Autodesk Inventor part; units mm, degrees
(part 2 of 3)
  line L420 (-40.5392, 1.7059) -> (-40.4752, 1.693) construction
  line L421 (-40.4117, 1.6779) -> (-40.3487, 1.6594) construction
  line L422 (-40.3487, 1.6594) -> (-40.2906, 1.6288) construction
  arc A72 (-40.2906, 1.6288) -> (-40.3121, 0.9596) centre (0, 0) ccw
  arc A73 (-40.3121, 0.9596) -> (-40.3225, 0.2901) centre (0, 0) ccw
  spline S135 degree 4 poles (-40.5744, 0.225) (-40.5099, 0.2348) (-40.4457, 0.2469) (-40.382, 0.2624) (-40.3225, 0.2901) knots 1 1 1 1 1 2 2 2 2 2
  line L423 (-40.5744, 0.225) -> (-40.5099, 0.2348) construction
  line L424 (-40.5099, 0.2348) -> (-40.4457, 0.2469) construction
  line L425 (-40.4457, 0.2469) -> (-40.382, 0.2624) construction
  line L426 (-40.382, 0.2624) -> (-40.3225, 0.2901) construction
  line L427 (-42.9441, -4.507) -> (-41.7202, -3.9838) construction
  spline S136 degree 2 poles (-42.9441, -4.507) (-41.7202, -3.9838) (-40.4121, -3.6329) knots 1 1 1 2 2 2
  line L428 (-41.7202, -3.9838) -> (-40.4121, -3.6329) construction
  spline S137 degree 2 poles (-43.1484, -1.6505) (-41.8625, -1.9942) (-40.5178, -2.1553) knots 1 1 1 2 2 2
  line L429 (-43.1484, -1.6505) -> (-41.8625, -1.9942) construction
  line L430 (-41.8625, -1.9942) -> (-40.5178, -2.1553) construction
  line L431 (-40.4528, -2.1621) -> (-40.3882, -2.1711) construction
  spline S138 degree 4 poles (-40.5178, -2.1553) (-40.4528, -2.1621) (-40.3882, -2.1711) (-40.3237, -2.1835) (-40.263, -2.2084) knots 1 1 1 1 1 2 2 2 2 2
  line L432 (-40.5178, -2.1553) -> (-40.4528, -2.1621) construction
  line L433 (-40.3882, -2.1711) -> (-40.3237, -2.1835) construction
  line L434 (-40.3237, -2.1835) -> (-40.263, -2.2084) construction
  arc A74 (-40.263, -2.2084) -> (-40.2208, -2.8766) centre (0, 0) ccw
  arc A75 (-40.2208, -2.8766) -> (-40.1675, -3.5441) centre (0, 0) ccw
  spline S139 degree 4 poles (-40.4121, -3.6329) (-40.3488, -3.617) (-40.286, -3.5988) (-40.224, -3.5774) (-40.1675, -3.5441) knots 1 1 1 1 1 2 2 2 2 2
  line L435 (-40.4121, -3.6329) -> (-40.3488, -3.617) construction
  line L436 (-40.3488, -3.617) -> (-40.286, -3.5988) construction
  line L437 (-40.286, -3.5988) -> (-40.224, -3.5774) construction
  line L438 (-40.224, -3.5774) -> (-40.1675, -3.5441) construction
  line L439 (-42.3213, -8.5687) -> (-41.1526, -7.9315) construction
  spline S140 degree 2 poles (-42.3213, -8.5687) (-41.1526, -7.9315) (-39.8838, -7.4578) knots 1 1 1 2 2 2
  line L440 (-41.1526, -7.9315) -> (-39.8838, -7.4578) construction
  spline S141 degree 2 poles (-42.7962, -5.7445) (-41.4834, -5.9644) (-40.1294, -5.997) knots 1 1 1 2 2 2
  line L441 (-42.7962, -5.7445) -> (-41.4834, -5.9644) construction
  line L442 (-41.4834, -5.9644) -> (-40.1294, -5.997) construction
  line L443 (-40.0641, -5.9976) -> (-39.9989, -6.0004) construction
  spline S142 degree 4 poles (-40.1294, -5.997) (-40.0641, -5.9976) (-39.9989, -6.0004) (-39.9336, -6.0067) (-39.8708, -6.0257) knots 1 1 1 1 1 2 2 2 2 2
  line L444 (-40.1294, -5.997) -> (-40.0641, -5.9976) construction
  line L445 (-39.9989, -6.0004) -> (-39.9336, -6.0067) construction
  line L446 (-39.9336, -6.0067) -> (-39.8708, -6.0257) construction
  arc A76 (-39.8708, -6.0257) -> (-39.7652, -6.6869) centre (0, 0) ccw
  arc A77 (-39.7652, -6.6869) -> (-39.6487, -7.3462) centre (0, 0) ccw
  spline S143 degree 4 poles (-39.8838, -7.4578) (-39.8223, -7.436) (-39.7615, -7.412) (-39.7019, -7.3847) (-39.6487, -7.3462) knots 1 1 1 1 1 2 2 2 2 2
  line L447 (-39.8838, -7.4578) -> (-39.8223, -7.436) construction
  line L448 (-39.8223, -7.436) -> (-39.7615, -7.412) construction
  line L449 (-39.7615, -7.412) -> (-39.7019, -7.3847) construction
  line L450 (-39.7019, -7.3847) -> (-39.6487, -7.3462) construction
  line L451 (-41.3151, -12.5528) -> (-40.2124, -11.8074) construction
  spline S144 degree 2 poles (-41.3151, -12.5528) (-40.2124, -11.8074) (-38.9943, -11.2153) knots 1 1 1 2 2 2
  line L452 (-40.2124, -11.8074) -> (-38.9943, -11.2153) construction
  spline S145 degree 2 poles (-42.0563, -9.7866) (-40.7286, -9.8807) (-39.3777, -9.7844) knots 1 1 1 2 2 2
  line L453 (-42.0563, -9.7866) -> (-40.7286, -9.8807) construction
  line L454 (-40.7286, -9.8807) -> (-39.3777, -9.7844) construction
  line L455 (-39.3126, -9.7787) -> (-39.2474, -9.7754) construction
  spline S146 degree 4 poles (-39.3777, -9.7844) (-39.3126, -9.7787) (-39.2474, -9.7754) (-39.1818, -9.7754) (-39.1175, -9.7883) knots 1 1 1 1 1 2 2 2 2 2
  line L456 (-39.3777, -9.7844) -> (-39.3126, -9.7787) construction
  line L457 (-39.2474, -9.7754) -> (-39.1818, -9.7754) construction
  line L458 (-39.1818, -9.7754) -> (-39.1175, -9.7883) construction
  arc A78 (-39.1175, -9.7883) -> (-38.9496, -10.4365) centre (0, 0) ccw
  arc A79 (-38.9496, -10.4365) -> (-38.7709, -11.0818) centre (0, 0) ccw
  spline S147 degree 4 poles (-38.9943, -11.2153) (-38.9351, -11.1877) (-38.8769, -11.158) (-38.8201, -11.1252) (-38.7709, -11.0818) knots 1 1 1 1 1 2 2 2 2 2
  line L459 (-38.9943, -11.2153) -> (-38.9351, -11.1877) construction
  line L460 (-38.9351, -11.1877) -> (-38.8769, -11.158) construction
  line L461 (-38.8769, -11.158) -> (-38.8201, -11.1252) construction
  line L462 (-38.8201, -11.1252) -> (-38.7709, -11.0818) construction
  line L463 (-39.9348, -16.4232) -> (-38.9079, -15.5764) construction
  spline S148 degree 2 poles (-39.9348, -16.4232) (-38.9079, -15.5764) (-37.7516, -14.8711) knots 1 1 1 2 2 2
  line L464 (-38.9079, -15.5764) -> (-37.7516, -14.8711) construction
  spline S149 degree 2 poles (-40.9356, -13.7399) (-39.605, -13.7074) (-38.2693, -13.4832) knots 1 1 1 2 2 2
  line L465 (-40.9356, -13.7399) -> (-39.605, -13.7074) construction
  line L466 (-39.605, -13.7074) -> (-38.2693, -13.4832) construction
  line L467 (-38.2051, -13.4714) -> (-38.1405, -13.4618) construction
  spline S150 degree 4 poles (-38.2693, -13.4832) (-38.2051, -13.4714) (-38.1405, -13.4618) (-38.0752, -13.4556) (-38.0099, -13.4624) knots 1 1 1 1 1 2 2 2 2 2
  line L468 (-38.2693, -13.4832) -> (-38.2051, -13.4714) construction
  line L469 (-38.1405, -13.4618) -> (-38.0752, -13.4556) construction
  line L470 (-38.0752, -13.4556) -> (-38.0099, -13.4624) construction
  arc A80 (-38.0099, -13.4624) -> (-37.7811, -14.0916) centre (0, 0) ccw
  arc A81 (-37.7811, -14.0916) -> (-37.5419, -14.717) centre (0, 0) ccw
  spline S151 degree 4 poles (-37.7516, -14.8711) (-37.6953, -14.838) (-37.6403, -14.8029) (-37.5868, -14.7649) (-37.5419, -14.717) knots 1 1 1 1 1 2 2 2 2 2
  line L471 (-37.7516, -14.8711) -> (-37.6953, -14.838) construction
  line L472 (-37.6953, -14.838) -> (-37.6403, -14.8029) construction
  line L473 (-37.6403, -14.8029) -> (-37.5868, -14.7649) construction
  line L474 (-37.5868, -14.7649) -> (-37.5419, -14.717) construction
  line L475 (-38.1929, -20.1449) -> (-37.2511, -19.2043) construction
  spline S152 degree 2 poles (-38.1929, -20.1449) (-37.2511, -19.2043) (-36.1671, -18.3923) knots 1 1 1 2 2 2
  line L476 (-37.2511, -19.2043) -> (-36.1671, -18.3923) construction
  spline S153 degree 2 poles (-39.4442, -17.5689) (-38.1227, -17.41) (-36.8144, -17.0599) knots 1 1 1 2 2 2
  line L477 (-39.4442, -17.5689) -> (-38.1227, -17.41) construction
  line L478 (-38.1227, -17.41) -> (-36.8144, -17.0599) construction
  line L479 (-36.7515, -17.042) -> (-36.6882, -17.0263) construction
  spline S154 degree 4 poles (-36.8144, -17.0599) (-36.7515, -17.042) (-36.6882, -17.0263) (-36.6237, -17.0139) (-36.5581, -17.0145) knots 1 1 1 1 1 2 2 2 2 2
  line L480 (-36.8144, -17.0599) -> (-36.7515, -17.042) construction
  line L481 (-36.6882, -17.0263) -> (-36.6237, -17.0139) construction
  line L482 (-36.6237, -17.0139) -> (-36.5581, -17.0145) construction
  arc A82 (-36.5581, -17.0145) -> (-36.2706, -17.6192) centre (0, 0) ccw
  arc A83 (-36.2706, -17.6192) -> (-35.973, -18.219) centre (0, 0) ccw
  spline S155 degree 4 poles (-36.1671, -18.3923) (-36.1142, -18.354) (-36.0627, -18.3138) (-36.0131, -18.2709) (-35.973, -18.219) knots 1 1 1 1 1 2 2 2 2 2
  line L483 (-36.1671, -18.3923) -> (-36.1142, -18.354) construction
  line L484 (-36.1142, -18.354) -> (-36.0627, -18.3138) construction
  line L485 (-36.0627, -18.3138) -> (-36.0131, -18.2709) construction
  line L486 (-36.0131, -18.2709) -> (-35.973, -18.219) construction
  line L487 (-36.1051, -23.6841) -> (-35.2569, -22.6583) construction
  spline S156 degree 2 poles (-36.1051, -23.6841) (-35.2569, -22.6583) (-34.255, -21.7469) knots 1 1 1 2 2 2
  line L488 (-35.2569, -22.6583) -> (-34.255, -21.7469) construction
  spline S157 degree 2 poles (-37.5956, -21.2388) (-36.2951, -20.955) (-35.026, -20.4821) knots 1 1 1 2 2 2
  line L489 (-37.5956, -21.2388) -> (-36.2951, -20.955) construction
  line L490 (-36.2951, -20.955) -> (-35.026, -20.4821) construction
  line L491 (-34.9652, -20.4583) -> (-34.9036, -20.4367) construction
  spline S158 degree 4 poles (-35.026, -20.4821) (-34.9652, -20.4583) (-34.9036, -20.4367) (-34.8406, -20.4182) (-34.7752, -20.4125) knots 1 1 1 1 1 2 2 2 2 2
  line L492 (-35.026, -20.4821) -> (-34.9652, -20.4583) construction
  line L493 (-34.9036, -20.4367) -> (-34.8406, -20.4182) construction
  line L494 (-34.8406, -20.4182) -> (-34.7752, -20.4125) construction
  arc A84 (-34.7752, -20.4125) -> (-34.4315, -20.9871) centre (0, 0) ccw
  arc A85 (-34.4315, -20.9871) -> (-34.0783, -21.5559) centre (0, 0) ccw
  spline S159 degree 4 poles (-34.255, -21.7469) (-34.206, -21.7038) (-34.1586, -21.6589) (-34.1133, -21.6114) (-34.0783, -21.5559) knots 1 1 1 1 1 2 2 2 2 2
  line L495 (-34.255, -21.7469) -> (-34.206, -21.7038) construction
  line L496 (-34.206, -21.7038) -> (-34.1586, -21.6589) construction
  line L497 (-34.1586, -21.6589) -> (-34.1133, -21.6114) construction
  line L498 (-34.1133, -21.6114) -> (-34.0783, -21.5559) construction
  line L499 (-33.6903, -27.0089) -> (-32.9435, -25.907) construction
  spline S160 degree 2 poles (-33.6903, -27.0089) (-32.9435, -25.907) (-32.0327, -24.9046) knots 1 1 1 2 2 2
  line L500 (-32.9435, -25.907) -> (-32.0327, -24.9046) construction
  spline S161 degree 2 poles (-35.4065, -24.7163) (-34.1389, -24.3102) (-32.9205, -23.7188) knots 1 1 1 2 2 2
  line L501 (-35.4065, -24.7163) -> (-34.1389, -24.3102) construction
  line L502 (-34.1389, -24.3102) -> (-32.9205, -23.7188) construction
  line L503 (-32.8622, -23.6893) -> (-32.8029, -23.6619) construction
  spline S162 degree 4 poles (-32.9205, -23.7188) (-32.8622, -23.6893) (-32.8029, -23.6619) (-32.742, -23.6376) (-32.6774, -23.6257) knots 1 1 1 1 1 2 2 2 2 2
  line L504 (-32.9205, -23.7188) -> (-32.8622, -23.6893) construction
  line L505 (-32.8029, -23.6619) -> (-32.742, -23.6376) construction
  line L506 (-32.742, -23.6376) -> (-32.6774, -23.6257) construction
  arc A86 (-32.6774, -23.6257) -> (-32.2807, -24.165) centre (0, 0) ccw
  arc A87 (-32.2807, -24.165) -> (-31.875, -24.6977) centre (0, 0) ccw
  spline S163 degree 4 poles (-32.0327, -24.9046) (-31.9881, -24.857) (-31.9451, -24.8078) (-31.9046, -24.7562) (-31.875, -24.6977) knots 1 1 1 1 1 2 2 2 2 2
  line L507 (-32.0327, -24.9046) -> (-31.9881, -24.857) construction
  line L508 (-31.9881, -24.857) -> (-31.9451, -24.8078) construction
  line L509 (-31.9451, -24.8078) -> (-31.9046, -24.7562) construction
  line L510 (-31.9046, -24.7562) -> (-31.875, -24.6977) construction
  line L511 (-30.9703, -30.089) -> (-30.3317, -28.9212) construction
  spline S164 degree 2 poles (-30.9703, -30.089) (-30.3317, -28.9212) (-29.5204, -27.8367) knots 1 1 1 2 2 2
  line L512 (-30.3317, -28.9212) -> (-29.5204, -27.8367) construction
  spline S165 degree 2 poles (-32.8967, -27.97) (-31.6735, -27.4452) (-30.5168, -26.7406) knots 1 1 1 2 2 2
  line L513 (-32.8967, -27.97) -> (-31.6735, -27.4452) construction
  line L514 (-31.6735, -27.4452) -> (-30.5168, -26.7406) construction
  line L515 (-30.4616, -26.7058) -> (-30.4051, -26.6729) construction
  spline S166 degree 4 poles (-30.5168, -26.7406) (-30.4616, -26.7058) (-30.4051, -26.6729) (-30.3468, -26.6429) (-30.2837, -26.6249) knots 1 1 1 1 1 2 2 2 2 2
  line L516 (-30.5168, -26.7406) -> (-30.4616, -26.7058) construction
  line L517 (-30.4051, -26.6729) -> (-30.3468, -26.6429) construction
  line L518 (-30.3468, -26.6429) -> (-30.2837, -26.6249) construction
  arc A88 (-30.2837, -26.6249) -> (-29.8375, -27.1241) centre (0, 0) ccw
  arc A89 (-29.8375, -27.1241) -> (-29.383, -27.6157) centre (0, 0) ccw
  spline S167 degree 4 poles (-29.5204, -27.8367) (-29.4804, -27.7851) (-29.4423, -27.732) (-29.4069, -27.6768) (-29.383, -27.6157) knots 1 1 1 1 1 2 2 2 2 2
  line L519 (-29.5204, -27.8367) -> (-29.4804, -27.7851) construction
  line L520 (-29.4804, -27.7851) -> (-29.4423, -27.732) construction
  line L521 (-29.4423, -27.732) -> (-29.4069, -27.6768) construction
  line L522 (-29.4069, -27.6768) -> (-29.383, -27.6157) construction
  line L523 (-27.97, -32.8967) -> (-27.4452, -31.6735) construction
  spline S168 degree 2 poles (-27.97, -32.8967) (-27.4452, -31.6735) (-26.7406, -30.5168) knots 1 1 1 2 2 2
  line L524 (-27.4452, -31.6735) -> (-26.7406, -30.5168) construction
  spline S169 degree 2 poles (-30.089, -30.9703) (-28.9212, -30.3317) (-27.8367, -29.5204) knots 1 1 1 2 2 2
  line L525 (-30.089, -30.9703) -> (-28.9212, -30.3317) construction
  line L526 (-28.9212, -30.3317) -> (-27.8367, -29.5204) construction
  line L527 (-27.7851, -29.4804) -> (-27.732, -29.4423) construction
  spline S170 degree 4 poles (-27.8367, -29.5204) (-27.7851, -29.4804) (-27.732, -29.4423) (-27.6768, -29.4069) (-27.6157, -29.383) knots 1 1 1 1 1 2 2 2 2 2
  line L528 (-27.8367, -29.5204) -> (-27.7851, -29.4804) construction
  line L529 (-27.732, -29.4423) -> (-27.6768, -29.4069) construction
  line L530 (-27.6768, -29.4069) -> (-27.6157, -29.383) construction
  arc A90 (-27.6157, -29.383) -> (-27.1241, -29.8375) centre (0, 0) ccw
  arc A91 (-27.1241, -29.8375) -> (-26.6249, -30.2837) centre (0, 0) ccw
  spline S171 degree 4 poles (-26.7406, -30.5168) (-26.7058, -30.4616) (-26.6729, -30.4051) (-26.6429, -30.3468) (-26.6249, -30.2837) knots 1 1 1 1 1 2 2 2 2 2
  line L531 (-26.7406, -30.5168) -> (-26.7058, -30.4616) construction
  line L532 (-26.7058, -30.4616) -> (-26.6729, -30.4051) construction
  line L533 (-26.6729, -30.4051) -> (-26.6429, -30.3468) construction
  line L534 (-26.6429, -30.3468) -> (-26.6249, -30.2837) construction
  line L535 (-24.7163, -35.4065) -> (-24.3102, -34.1389) construction
  spline S172 degree 2 poles (-24.7163, -35.4065) (-24.3102, -34.1389) (-23.7188, -32.9205) knots 1 1 1 2 2 2
  line L536 (-24.3102, -34.1389) -> (-23.7188, -32.9205) construction
  spline S173 degree 2 poles (-27.0089, -33.6903) (-25.907, -32.9435) (-24.9046, -32.0327) knots 1 1 1 2 2 2
  line L537 (-27.0089, -33.6903) -> (-25.907, -32.9435) construction
  line L538 (-25.907, -32.9435) -> (-24.9046, -32.0327) construction
  line L539 (-24.857, -31.9881) -> (-24.8078, -31.9451) construction
  spline S174 degree 4 poles (-24.9046, -32.0327) (-24.857, -31.9881) (-24.8078, -31.9451) (-24.7562, -31.9046) (-24.6977, -31.875) knots 1 1 1 1 1 2 2 2 2 2
  line L540 (-24.9046, -32.0327) -> (-24.857, -31.9881) construction
  line L541 (-24.8078, -31.9451) -> (-24.7562, -31.9046) construction
  line L542 (-24.7562, -31.9046) -> (-24.6977, -31.875) construction
  arc A92 (-24.6977, -31.875) -> (-24.165, -32.2807) centre (0, 0) ccw
  arc A93 (-24.165, -32.2807) -> (-23.6257, -32.6774) centre (0, 0) ccw
  spline S175 degree 4 poles (-23.7188, -32.9205) (-23.6893, -32.8622) (-23.6619, -32.8029) (-23.6376, -32.742) (-23.6257, -32.6774) knots 1 1 1 1 1 2 2 2 2 2
  line L543 (-23.7188, -32.9205) -> (-23.6893, -32.8622) construction
  line L544 (-23.6893, -32.8622) -> (-23.6619, -32.8029) construction
  line L545 (-23.6619, -32.8029) -> (-23.6376, -32.742) construction
  line L546 (-23.6376, -32.742) -> (-23.6257, -32.6774) construction
  line L547 (-21.2388, -37.5956) -> (-20.955, -36.2951) construction
  spline S176 degree 2 poles (-21.2388, -37.5956) (-20.955, -36.2951) (-20.4821, -35.026) knots 1 1 1 2 2 2
  line L548 (-20.955, -36.2951) -> (-20.4821, -35.026) construction
  spline S177 degree 2 poles (-23.6841, -36.1051) (-22.6583, -35.2569) (-21.7469, -34.255) knots 1 1 1 2 2 2
  line L549 (-23.6841, -36.1051) -> (-22.6583, -35.2569) construction
  line L550 (-22.6583, -35.2569) -> (-21.7469, -34.255) construction
  line L551 (-21.7038, -34.206) -> (-21.6589, -34.1586) construction
  spline S178 degree 4 poles (-21.7469, -34.255) (-21.7038, -34.206) (-21.6589, -34.1586) (-21.6114, -34.1133) (-21.5559, -34.0783) knots 1 1 1 1 1 2 2 2 2 2
  line L552 (-21.7469, -34.255) -> (-21.7038, -34.206) construction
  line L553 (-21.6589, -34.1586) -> (-21.6114, -34.1133) construction
  line L554 (-21.6114, -34.1133) -> (-21.5559, -34.0783) construction
  arc A94 (-21.5559, -34.0783) -> (-20.9871, -34.4315) centre (0, 0) ccw
  arc A95 (-20.9871, -34.4315) -> (-20.4125, -34.7752) centre (0, 0) ccw
  spline S179 degree 4 poles (-20.4821, -35.026) (-20.4583, -34.9652) (-20.4367, -34.9036) (-20.4182, -34.8406) (-20.4125, -34.7752) knots 1 1 1 1 1 2 2 2 2 2
  line L555 (-20.4821, -35.026) -> (-20.4583, -34.9652) construction
  line L556 (-20.4583, -34.9652) -> (-20.4367, -34.9036) construction
  line L557 (-20.4367, -34.9036) -> (-20.4182, -34.8406) construction
  line L558 (-20.4182, -34.8406) -> (-20.4125, -34.7752) construction
  line L559 (-17.5689, -39.4442) -> (-17.41, -38.1227) construction
  spline S180 degree 2 poles (-17.5689, -39.4442) (-17.41, -38.1227) (-17.0599, -36.8144) knots 1 1 1 2 2 2
  line L560 (-17.41, -38.1227) -> (-17.0599, -36.8144) construction
  spline S181 degree 2 poles (-20.1449, -38.1929) (-19.2043, -37.2511) (-18.3923, -36.1671) knots 1 1 1 2 2 2
  line L561 (-20.1449, -38.1929) -> (-19.2043, -37.2511) construction
  line L562 (-19.2043, -37.2511) -> (-18.3923, -36.1671) construction
  line L563 (-18.354, -36.1142) -> (-18.3138, -36.0627) construction
  spline S182 degree 4 poles (-18.3923, -36.1671) (-18.354, -36.1142) (-18.3138, -36.0627) (-18.2709, -36.0131) (-18.219, -35.973) knots 1 1 1 1 1 2 2 2 2 2
  line L564 (-18.3923, -36.1671) -> (-18.354, -36.1142) construction
  line L565 (-18.3138, -36.0627) -> (-18.2709, -36.0131) construction
  line L566 (-18.2709, -36.0131) -> (-18.219, -35.973) construction
  arc A96 (-18.219, -35.973) -> (-17.6192, -36.2706) centre (0, 0) ccw
  arc A97 (-17.6192, -36.2706) -> (-17.0145, -36.5581) centre (0, 0) ccw
  spline S183 degree 4 poles (-17.0599, -36.8144) (-17.042, -36.7515) (-17.0263, -36.6882) (-17.0139, -36.6237) (-17.0145, -36.5581) knots 1 1 1 1 1 2 2 2 2 2
  line L567 (-17.0599, -36.8144) -> (-17.042, -36.7515) construction
  line L568 (-17.042, -36.7515) -> (-17.0263, -36.6882) construction
  line L569 (-17.0263, -36.6882) -> (-17.0139, -36.6237) construction
  line L570 (-17.0139, -36.6237) -> (-17.0145, -36.5581) construction
  line L571 (-13.7399, -40.9356) -> (-13.7074, -39.605) construction
  spline S184 degree 2 poles (-13.7399, -40.9356) (-13.7074, -39.605) (-13.4832, -38.2693) knots 1 1 1 2 2 2
  line L572 (-13.7074, -39.605) -> (-13.4832, -38.2693) construction
  spline S185 degree 2 poles (-16.4232, -39.9348) (-15.5764, -38.9079) (-14.8711, -37.7516) knots 1 1 1 2 2 2
  line L573 (-16.4232, -39.9348) -> (-15.5764, -38.9079) construction
  line L574 (-15.5764, -38.9079) -> (-14.8711, -37.7516) construction
  line L575 (-14.838, -37.6953) -> (-14.8029, -37.6403) construction
  spline S186 degree 4 poles (-14.8711, -37.7516) (-14.838, -37.6953) (-14.8029, -37.6403) (-14.7649, -37.5868) (-14.717, -37.5419) knots 1 1 1 1 1 2 2 2 2 2
  line L576 (-14.8711, -37.7516) -> (-14.838, -37.6953) construction
  line L577 (-14.8029, -37.6403) -> (-14.7649, -37.5868) construction
  line L578 (-14.7649, -37.5868) -> (-14.717, -37.5419) construction
  arc A98 (-14.717, -37.5419) -> (-14.0916, -37.7811) centre (0, 0) ccw
  arc A99 (-14.0916, -37.7811) -> (-13.4624, -38.0099) centre (0, 0) ccw
  spline S187 degree 4 poles (-13.4832, -38.2693) (-13.4714, -38.2051) (-13.4618, -38.1405) (-13.4556, -38.0752) (-13.4624, -38.0099) knots 1 1 1 1 1 2 2 2 2 2
  line L579 (-13.4832, -38.2693) -> (-13.4714, -38.2051) construction
  line L580 (-13.4714, -38.2051) -> (-13.4618, -38.1405) construction
  line L581 (-13.4618, -38.1405) -> (-13.4556, -38.0752) construction
  line L582 (-13.4556, -38.0752) -> (-13.4624, -38.0099) construction
  line L583 (-9.7866, -42.0563) -> (-9.8807, -40.7286) construction
  spline S188 degree 2 poles (-9.7866, -42.0563) (-9.8807, -40.7286) (-9.7844, -39.3777) knots 1 1 1 2 2 2
  line L584 (-9.8807, -40.7286) -> (-9.7844, -39.3777) construction
  spline S189 degree 2 poles (-12.5528, -41.3151) (-11.8074, -40.2124) (-11.2153, -38.9943) knots 1 1 1 2 2 2
  line L585 (-12.5528, -41.3151) -> (-11.8074, -40.2124) construction
  line L586 (-11.8074, -40.2124) -> (-11.2153, -38.9943) construction
  line L587 (-11.1877, -38.9351) -> (-11.158, -38.8769) construction
  spline S190 degree 4 poles (-11.2153, -38.9943) (-11.1877, -38.9351) (-11.158, -38.8769) (-11.1252, -38.8201) (-11.0818, -38.7709) knots 1 1 1 1 1 2 2 2 2 2
  line L588 (-11.2153, -38.9943) -> (-11.1877, -38.9351) construction
  line L589 (-11.158, -38.8769) -> (-11.1252, -38.8201) construction
  line L590 (-11.1252, -38.8201) -> (-11.0818, -38.7709) construction
  arc A100 (-11.0818, -38.7709) -> (-10.4365, -38.9496) centre (0, 0) ccw
  arc A101 (-10.4365, -38.9496) -> (-9.7883, -39.1175) centre (0, 0) ccw
  spline S191 degree 4 poles (-9.7844, -39.3777) (-9.7787, -39.3126) (-9.7754, -39.2474) (-9.7754, -39.1818) (-9.7883, -39.1175) knots 1 1 1 1 1 2 2 2 2 2
  line L591 (-9.7844, -39.3777) -> (-9.7787, -39.3126) construction
  line L592 (-9.7787, -39.3126) -> (-9.7754, -39.2474) construction
  line L593 (-9.7754, -39.2474) -> (-9.7754, -39.1818) construction
  line L594 (-9.7754, -39.1818) -> (-9.7883, -39.1175) construction
  line L595 (-5.7445, -42.7962) -> (-5.9644, -41.4834) construction
  spline S192 degree 2 poles (-5.7445, -42.7962) (-5.9644, -41.4834) (-5.997, -40.1294) knots 1 1 1 2 2 2
  line L596 (-5.9644, -41.4834) -> (-5.997, -40.1294) construction
  spline S193 degree 2 poles (-8.5687, -42.3213) (-7.9315, -41.1526) (-7.4578, -39.8838) knots 1 1 1 2 2 2
  line L597 (-8.5687, -42.3213) -> (-7.9315, -41.1526) construction
  line L598 (-7.9315, -41.1526) -> (-7.4578, -39.8838) construction
  line L599 (-7.436, -39.8223) -> (-7.412, -39.7615) construction
  spline S194 degree 4 poles (-7.4578, -39.8838) (-7.436, -39.8223) (-7.412, -39.7615) (-7.3847, -39.7019) (-7.3462, -39.6487) knots 1 1 1 1 1 2 2 2 2 2
  line L600 (-7.4578, -39.8838) -> (-7.436, -39.8223) construction
  line L601 (-7.412, -39.7615) -> (-7.3847, -39.7019) construction
  line L602 (-7.3847, -39.7019) -> (-7.3462, -39.6487) construction
  arc A102 (-7.3462, -39.6487) -> (-6.6869, -39.7652) centre (0, 0) ccw
  arc A103 (-6.6869, -39.7652) -> (-6.0257, -39.8708) centre (0, 0) ccw
  spline S195 degree 4 poles (-5.997, -40.1294) (-5.9976, -40.0641) (-6.0004, -39.9989) (-6.0067, -39.9336) (-6.0257, -39.8708) knots 1 1 1 1 1 2 2 2 2 2
  line L603 (-5.997, -40.1294) -> (-5.9976, -40.0641) construction
  line L604 (-5.9976, -40.0641) -> (-6.0004, -39.9989) construction
  line L605 (-6.0004, -39.9989) -> (-6.0067, -39.9336) construction
  line L606 (-6.0067, -39.9336) -> (-6.0257, -39.8708) construction
  line L607 (-1.6505, -43.1484) -> (-1.9942, -41.8625) construction
  spline S196 degree 2 poles (-1.6505, -43.1484) (-1.9942, -41.8625) (-2.1553, -40.5178) knots 1 1 1 2 2 2
  line L608 (-1.9942, -41.8625) -> (-2.1553, -40.5178) construction
  spline S197 degree 2 poles (-4.507, -42.9441) (-3.9838, -41.7202) (-3.6329, -40.4121) knots 1 1 1 2 2 2
  line L609 (-4.507, -42.9441) -> (-3.9838, -41.7202) construction
  line L610 (-3.9838, -41.7202) -> (-3.6329, -40.4121) construction
  line L611 (-3.617, -40.3488) -> (-3.5988, -40.286) construction
  spline S198 degree 4 poles (-3.6329, -40.4121) (-3.617, -40.3488) (-3.5988, -40.286) (-3.5774, -40.224) (-3.5441, -40.1675) knots 1 1 1 1 1 2 2 2 2 2
  line L612 (-3.6329, -40.4121) -> (-3.617, -40.3488) construction
  line L613 (-3.5988, -40.286) -> (-3.5774, -40.224) construction
  line L614 (-3.5774, -40.224) -> (-3.5441, -40.1675) construction
  arc A104 (-3.5441, -40.1675) -> (-2.8766, -40.2208) centre (0, 0) ccw
  arc A105 (-2.8766, -40.2208) -> (-2.2084, -40.263) centre (0, 0) ccw
  spline S199 degree 4 poles (-2.1553, -40.5178) (-2.1621, -40.4528) (-2.1711, -40.3882) (-2.1835, -40.3237) (-2.2084, -40.263) knots 1 1 1 1 1 2 2 2 2 2
  line L615 (-2.1553, -40.5178) -> (-2.1621, -40.4528) construction
  line L616 (-2.1621, -40.4528) -> (-2.1711, -40.3882) construction
  line L617 (-2.1711, -40.3882) -> (-2.1835, -40.3237) construction
  line L618 (-2.1835, -40.3237) -> (-2.2084, -40.263) construction
  line L619 (2.4585, -43.11) -> (1.9942, -41.8625) construction
  spline S200 degree 2 poles (2.4585, -43.11) (1.9942, -41.8625) (1.7059, -40.5392) knots 1 1 1 2 2 2
  line L620 (1.9942, -41.8625) -> (1.7059, -40.5392) construction
  spline S201 degree 2 poles (-0.4045, -43.1781) (0, -41.91) (0.225, -40.5744) knots 1 1 1 2 2 2
  line L621 (-0.4045, -43.1781) -> (0, -41.91) construction
  line L622 (0, -41.91) -> (0.225, -40.5744) construction
  line L623 (0.2348, -40.5099) -> (0.2469, -40.4457) construction
  spline S202 degree 4 poles (0.225, -40.5744) (0.2348, -40.5099) (0.2469, -40.4457) (0.2624, -40.382) (0.2901, -40.3225) knots 1 1 1 1 1 2 2 2 2 2
  line L624 (0.225, -40.5744) -> (0.2348, -40.5099) construction
  line L625 (0.2469, -40.4457) -> (0.2624, -40.382) construction
  line L626 (0.2624, -40.382) -> (0.2901, -40.3225) construction
  arc A106 (0.2901, -40.3225) -> (0.9596, -40.3121) centre (0, 0) ccw
  arc A107 (0.9596, -40.3121) -> (1.6288, -40.2906) centre (0, 0) ccw
  spline S203 degree 4 poles (1.7059, -40.5392) (1.693, -40.4752) (1.6779, -40.4117) (1.6594, -40.3487) (1.6288, -40.2906) knots 1 1 1 1 1 2 2 2 2 2
  line L627 (1.7059, -40.5392) -> (1.693, -40.4752) construction
  line L628 (1.693, -40.4752) -> (1.6779, -40.4117) construction
  line L629 (1.6779, -40.4117) -> (1.6594, -40.3487) construction
  line L630 (1.6594, -40.3487) -> (1.6288, -40.2906) construction
  line L631 (6.5452, -42.6811) -> (5.9644, -41.4834) construction
  spline S204 degree 2 poles (6.5452, -42.6811) (5.9644, -41.4834) (5.5517, -40.1935) knots 1 1 1 2 2 2
  line L632 (5.9644, -41.4834) -> (5.5517, -40.1935) construction
  spline S205 degree 2 poles (3.7017, -43.021) (3.9838, -41.7202) (4.0808, -40.3693) knots 1 1 1 2 2 2
  line L633 (3.7017, -43.021) -> (3.9838, -41.7202) construction
  line L634 (3.9838, -41.7202) -> (4.0808, -40.3693) construction
  line L635 (4.0844, -40.3041) -> (4.0904, -40.2391) construction
  spline S206 degree 4 poles (4.0808, -40.3693) (4.0844, -40.3041) (4.0904, -40.2391) (4.0997, -40.1742) (4.1217, -40.1123) knots 1 1 1 1 1 2 2 2 2 2
  line L636 (4.0808, -40.3693) -> (4.0844, -40.3041) construction
  line L637 (4.0904, -40.2391) -> (4.0997, -40.1742) construction
  line L638 (4.0997, -40.1742) -> (4.1217, -40.1123) construction
  arc A108 (4.1217, -40.1123) -> (4.7872, -40.0384) centre (0, 0) ccw
  arc A109 (4.7872, -40.0384) -> (5.4513, -39.9534) centre (0, 0) ccw
  spline S207 degree 4 poles (5.5517, -40.1935) (5.5328, -40.131) (5.5116, -40.0692) (5.4872, -40.0083) (5.4513, -39.9534) knots 1 1 1 1 1 2 2 2 2 2
  line L639 (5.5517, -40.1935) -> (5.5328, -40.131) construction
  line L640 (5.5328, -40.131) -> (5.5116, -40.0692) construction
  line L641 (5.5116, -40.0692) -> (5.4872, -40.0083) construction
  line L642 (5.4872, -40.0083) -> (5.4513, -39.9534) construction
  line L643 (10.5727, -41.8656) -> (9.8807, -40.7286) construction
  spline S208 degree 2 poles (10.5727, -41.8656) (9.8807, -40.7286) (9.3471, -39.4838) knots 1 1 1 2 2 2
  line L644 (9.8807, -40.7286) -> (9.3471, -39.4838) construction
  spline S209 degree 2 poles (7.7743, -42.4744) (7.9315, -41.1526) (7.8997, -39.7986) knots 1 1 1 2 2 2
  line L645 (7.7743, -42.4744) -> (7.9315, -41.1526) construction
  line L646 (7.9315, -41.1526) -> (7.8997, -39.7986) construction
  line L647 (7.8971, -39.7334) -> (7.8968, -39.6681) construction
  spline S210 degree 4 poles (7.8997, -39.7986) (7.8971, -39.7334) (7.8968, -39.6681) (7.9, -39.6025) (7.916, -39.5389) knots 1 1 1 1 1 2 2 2 2 2
  line L648 (7.8997, -39.7986) -> (7.8971, -39.7334) construction
  line L649 (7.8968, -39.6681) -> (7.9, -39.6025) construction
  line L650 (7.9, -39.6025) -> (7.916, -39.5389) construction
  arc A110 (7.916, -39.5389) -> (8.5714, -39.402) centre (0, 0) ccw
  arc A111 (8.5714, -39.402) -> (9.2244, -39.2543) centre (0, 0) ccw
  spline S211 degree 4 poles (9.3471, -39.4838) (9.3224, -39.4233) (9.2955, -39.3638) (9.2654, -39.3055) (9.2244, -39.2543) knots 1 1 1 1 1 2 2 2 2 2
  line L651 (9.3471, -39.4838) -> (9.3224, -39.4233) construction
  line L652 (9.3224, -39.4233) -> (9.2955, -39.3638) construction
  line L653 (9.2955, -39.3638) -> (9.2654, -39.3055) construction
  line L654 (9.2654, -39.3055) -> (9.2244, -39.2543) construction
  line L655 (14.5044, -40.6711) -> (13.7074, -39.605) construction
  spline S212 degree 2 poles (14.5044, -40.6711) (13.7074, -39.605) (13.058, -38.4165) knots 1 1 1 2 2 2
  line L656 (13.7074, -39.605) -> (13.058, -38.4165) construction
  spline S213 degree 2 poles (11.7766, -41.543) (11.8074, -40.2124) (11.647, -38.8675) knots 1 1 1 2 2 2
  line L657 (11.7766, -41.543) -> (11.8074, -40.2124) construction
  line L658 (11.8074, -40.2124) -> (11.647, -38.8675) construction
  line L659 (11.6382, -38.8028) -> (11.6318, -38.7378) construction
  spline S214 degree 4 poles (11.647, -38.8675) (11.6382, -38.8028) (11.6318, -38.7378) (11.6287, -38.6723) (11.6385, -38.6074) knots 1 1 1 1 1 2 2 2 2 2
  line L660 (11.647, -38.8675) -> (11.6382, -38.8028) construction
  line L661 (11.6318, -38.7378) -> (11.6287, -38.6723) construction
  line L662 (11.6287, -38.6723) -> (11.6385, -38.6074) construction
  arc A112 (11.6385, -38.6074) -> (12.278, -38.4088) centre (0, 0) ccw
  arc A113 (12.278, -38.4088) -> (12.914, -38.1997) centre (0, 0) ccw
  spline S215 degree 4 poles (13.058, -38.4165) (13.0276, -38.3587) (12.9952, -38.302) (12.9597, -38.2468) (12.914, -38.1997) knots 1 1 1 1 1 2 2 2 2 2
  line L663 (13.058, -38.4165) -> (13.0276, -38.3587) construction
  line L664 (13.0276, -38.3587) -> (12.9952, -38.302) construction
  line L665 (12.9952, -38.302) -> (12.9597, -38.2468) construction
  line L666 (12.9597, -38.2468) -> (12.914, -38.1997) construction
  line L667 (18.3048, -39.1082) -> (17.41, -38.1227) construction
  spline S216 degree 2 poles (18.3048, -39.1082) (17.41, -38.1227) (16.6506, -37.0013) knots 1 1 1 2 2 2
  line L668 (17.41, -38.1227) -> (16.6506, -37.0013) construction
  spline S217 degree 2 poles (15.6722, -40.2355) (15.5764, -38.9079) (15.2889, -37.5844) knots 1 1 1 2 2 2
  line L669 (15.6722, -40.2355) -> (15.5764, -38.9079) construction
  line L670 (15.5764, -38.9079) -> (15.2889, -37.5844) construction
  line L671 (15.274, -37.5208) -> (15.2614, -37.4567) construction
  spline S218 degree 4 poles (15.2889, -37.5844) (15.274, -37.5208) (15.2614, -37.4567) (15.252, -37.3918) (15.2557, -37.3263) knots 1 1 1 1 1 2 2 2 2 2
  line L672 (15.2889, -37.5844) -> (15.274, -37.5208) construction
  line L673 (15.2614, -37.4567) -> (15.252, -37.3918) construction
  line L674 (15.252, -37.3918) -> (15.2557, -37.3263) construction
  arc A114 (15.2557, -37.3263) -> (15.8734, -37.0678) centre (0, 0) ccw
  arc A115 (15.8734, -37.0678) -> (16.4867, -36.7992) centre (0, 0) ccw
  spline S219 degree 4 poles (16.6506, -37.0013) (16.6148, -36.9466) (16.5772, -36.8933) (16.5366, -36.8417) (16.4867, -36.7992) knots 1 1 1 1 1 2 2 2 2 2
  line L675 (16.6506, -37.0013) -> (16.6148, -36.9466) construction
  line L676 (16.6148, -36.9466) -> (16.5772, -36.8933) construction
  line L677 (16.5772, -36.8933) -> (16.5366, -36.8417) construction
  line L678 (16.5366, -36.8417) -> (16.4867, -36.7992) construction
  line L679 (21.9393, -37.1911) -> (20.955, -36.2951) construction
  spline S220 degree 2 poles (21.9393, -37.1911) (20.955, -36.2951) (20.0924, -35.251) knots 1 1 1 2 2 2
  line L680 (20.955, -36.2951) -> (20.0924, -35.251) construction
  spline S221 degree 2 poles (19.4258, -38.5636) (19.2043, -37.2511) (18.7923, -35.9609) knots 1 1 1 2 2 2
  line L681 (19.4258, -38.5636) -> (19.2043, -37.2511) construction
  line L682 (19.2043, -37.2511) -> (18.7923, -35.9609) construction
  line L683 (18.7714, -35.899) -> (18.7528, -35.8364) construction
  spline S222 degree 4 poles (18.7923, -35.9609) (18.7714, -35.899) (18.7528, -35.8364) (18.7373, -35.7727) (18.7347, -35.7071) knots 1 1 1 1 1 2 2 2 2 2
  line L684 (18.7923, -35.9609) -> (18.7714, -35.899) construction
  line L685 (18.7528, -35.8364) -> (18.7373, -35.7727) construction
  line L686 (18.7373, -35.7727) -> (18.7347, -35.7071) construction
  arc A116 (18.7347, -35.7071) -> (19.325, -35.3911) centre (0, 0) ccw
  arc A117 (19.325, -35.3911) -> (19.91, -35.0654) centre (0, 0) ccw
  spline S223 degree 4 poles (20.0924, -35.251) (20.0516, -35.2) (20.009, -35.1505) (19.9637, -35.103) (19.91, -35.0654) knots 1 1 1 1 1 2 2 2 2 2
  line L687 (20.0924, -35.251) -> (20.0516, -35.2) construction
  line L688 (20.0516, -35.2) -> (20.009, -35.1505) construction
  line L689 (20.009, -35.1505) -> (19.9637, -35.103) construction
  line L690 (19.9637, -35.103) -> (19.91, -35.0654) construction
  line L691 (25.3752, -34.9372) -> (24.3102, -34.1389) construction
  spline S224 degree 2 poles (25.3752, -34.9372) (24.3102, -34.1389) (23.3522, -33.1815) knots 1 1 1 2 2 2
  line L692 (24.3102, -34.1389) -> (23.3522, -33.1815) construction
  spline S225 degree 2 poles (23.0036, -36.5424) (22.6583, -35.2569) (22.1255, -34.0118) knots 1 1 1 2 2 2
  line L693 (23.0036, -36.5424) -> (22.6583, -35.2569) construction
  line L694 (22.6583, -35.2569) -> (22.1255, -34.0118) construction
  line L695 (22.0988, -33.9521) -> (22.0743, -33.8916) construction
  spline S226 degree 4 poles (22.1255, -34.0118) (22.0988, -33.9521) (22.0743, -33.8916) (22.0529, -33.8296) (22.0441, -33.7646) knots 1 1 1 1 1 2 2 2 2 2
  line L696 (22.1255, -34.0118) -> (22.0988, -33.9521) construction
  line L697 (22.0743, -33.8916) -> (22.0529, -33.8296) construction
  line L698 (22.0529, -33.8296) -> (22.0441, -33.7646) construction
  arc A118 (22.0441, -33.7646) -> (22.6017, -33.3939) centre (0, 0) ccw
  arc A119 (22.6017, -33.3939) -> (23.153, -33.014) centre (0, 0) ccw
  spline S227 degree 4 poles (23.3522, -33.1815) (23.3068, -33.1346) (23.2597, -33.0893) (23.2101, -33.0464) (23.153, -33.014) knots 1 1 1 1 1 2 2 2 2 2
  line L699 (23.3522, -33.1815) -> (23.3068, -33.1346) construction
  line L700 (23.3068, -33.1346) -> (23.2597, -33.0893) construction
  line L701 (23.2597, -33.0893) -> (23.2101, -33.0464) construction
  line L702 (23.2101, -33.0464) -> (23.153, -33.014) construction
  line L703 (28.5813, -32.367) -> (27.4452, -31.6735) construction
  spline S228 degree 2 poles (28.5813, -32.367) (27.4452, -31.6735) (26.4006, -30.8115) knots 1 1 1 2 2 2
  line L704 (27.4452, -31.6735) -> (26.4006, -30.8115) construction
  spline S229 degree 2 poles (26.373, -34.1903) (25.907, -32.9435) (25.2583, -31.7546) knots 1 1 1 2 2 2
  line L705 (26.373, -34.1903) -> (25.907, -32.9435) construction
  line L706 (25.907, -32.9435) -> (25.2583, -31.7546) construction
  line L707 (25.2261, -31.6978) -> (25.196, -31.6399) construction
  spline S230 degree 4 poles (25.2583, -31.7546) (25.2261, -31.6978) (25.196, -31.6399) (25.1687, -31.5802) (25.1538, -31.5163) knots 1 1 1 1 1 2 2 2 2 2
  line L708 (25.2583, -31.7546) -> (25.2261, -31.6978) construction
  line L709 (25.196, -31.6399) -> (25.1687, -31.5802) construction
  line L710 (25.1687, -31.5802) -> (25.1538, -31.5163) construction
  arc A120 (25.1538, -31.5163) -> (25.6736, -31.0943) centre (0, 0) ccw
  arc A121 (25.6736, -31.0943) -> (26.1864, -30.6637) centre (0, 0) ccw
  spline S231 degree 4 poles (26.4006, -30.8115) (26.3509, -30.7691) (26.2997, -30.7285) (26.2463, -30.6905) (26.1864, -30.6637) knots 1 1 1 1 1 2 2 2 2 2
  line L711 (26.4006, -30.8115) -> (26.3509, -30.7691) construction
  line L712 (26.3509, -30.7691) -> (26.2997, -30.7285) construction
  line L713 (26.2997, -30.7285) -> (26.2463, -30.6905) construction
  line L714 (26.2463, -30.6905) -> (26.1864, -30.6637) construction
  line L715 (31.5286, -29.5036) -> (30.3317, -28.9212) construction
  spline S232 degree 2 poles (31.5286, -29.5036) (30.3317, -28.9212) (29.2099, -28.1624) knots 1 1 1 2 2 2
  line L716 (30.3317, -28.9212) -> (29.2099, -28.1624) construction
  spline S233 degree 2 poles (29.5036, -31.5286) (28.9212, -30.3317) (28.1624, -29.2099) knots 1 1 1 2 2 2
  line L717 (29.5036, -31.5286) -> (28.9212, -30.3317) construction
  line L718 (28.9212, -30.3317) -> (28.1624, -29.2099) construction
  line L719 (28.125, -29.1564) -> (28.0894, -29.1016) construction
  spline S234 degree 4 poles (28.1624, -29.2099) (28.125, -29.1564) (28.0894, -29.1016) (28.0566, -29.0447) (28.0357, -28.9825) knots 1 1 1 1 1 2 2 2 2 2
  line L720 (28.1624, -29.2099) -> (28.125, -29.1564) construction
  line L721 (28.0894, -29.1016) -> (28.0566, -29.0447) construction
  line L722 (28.0566, -29.0447) -> (28.0357, -28.9825) construction
  arc A122 (28.0357, -28.9825) -> (28.5131, -28.5131) centre (0, 0) ccw
  arc A123 (28.5131, -28.5131) -> (28.9825, -28.0357) centre (0, 0) ccw
  spline S235 degree 4 poles (29.2099, -28.1624) (29.1564, -28.125) (29.1016, -28.0894) (29.0447, -28.0566) (28.9825, -28.0357) knots 1 1 1 1 1 2 2 2 2 2
  line L723 (29.2099, -28.1624) -> (29.1564, -28.125) construction
  line L724 (29.1564, -28.125) -> (29.1016, -28.0894) construction
  line L725 (29.1016, -28.0894) -> (29.0447, -28.0566) construction
  line L726 (29.0447, -28.0566) -> (28.9825, -28.0357) construction
  line L727 (34.1903, -26.373) -> (32.9435, -25.907) construction
  spline S236 degree 2 poles (34.1903, -26.373) (32.9435, -25.907) (31.7546, -25.2583) knots 1 1 1 2 2 2
  line L728 (32.9435, -25.907) -> (31.7546, -25.2583) construction
  spline S237 degree 2 poles (32.367, -28.5813) (31.6735, -27.4452) (30.8115, -26.4006) knots 1 1 1 2 2 2
  line L729 (32.367, -28.5813) -> (31.6735, -27.4452) construction
  line L730 (31.6735, -27.4452) -> (30.8115, -26.4006) construction
  line L731 (30.7691, -26.3509) -> (30.7285, -26.2997) construction
  spline S238 degree 4 poles (30.8115, -26.4006) (30.7691, -26.3509) (30.7285, -26.2997) (30.6905, -26.2463) (30.6637, -26.1864) knots 1 1 1 1 1 2 2 2 2 2
  line L732 (30.8115, -26.4006) -> (30.7691, -26.3509) construction
  line L733 (30.7285, -26.2997) -> (30.6905, -26.2463) construction
  line L734 (30.6905, -26.2463) -> (30.6637, -26.1864) construction
  arc A124 (30.6637, -26.1864) -> (31.0943, -25.6736) centre (0, 0) ccw
  arc A125 (31.0943, -25.6736) -> (31.5163, -25.1538) centre (0, 0) ccw
  spline S239 degree 4 poles (31.7546, -25.2583) (31.6978, -25.2261) (31.6399, -25.196) (31.5802, -25.1687) (31.5163, -25.1538) knots 1 1 1 1 1 2 2 2 2 2
  line L735 (31.7546, -25.2583) -> (31.6978, -25.2261) construction
  line L736 (31.6978, -25.2261) -> (31.6399, -25.196) construction
  line L737 (31.6399, -25.196) -> (31.5802, -25.1687) construction
  line L738 (31.5802, -25.1687) -> (31.5163, -25.1538) construction
  line L739 (36.5424, -23.0036) -> (35.2569, -22.6583) construction
  spline S240 degree 2 poles (36.5424, -23.0036) (35.2569, -22.6583) (34.0118, -22.1255) knots 1 1 1 2 2 2
  line L740 (35.2569, -22.6583) -> (34.0118, -22.1255) construction
  spline S241 degree 2 poles (34.9372, -25.3752) (34.1389, -24.3102) (33.1815, -23.3522) knots 1 1 1 2 2 2
  line L741 (34.9372, -25.3752) -> (34.1389, -24.3102) construction
  line L742 (34.1389, -24.3102) -> (33.1815, -23.3522) construction
  line L743 (33.1346, -23.3068) -> (33.0893, -23.2597) construction
  spline S242 degree 4 poles (33.1815, -23.3522) (33.1346, -23.3068) (33.0893, -23.2597) (33.0464, -23.2101) (33.014, -23.153) knots 1 1 1 1 1 2 2 2 2 2
  line L744 (33.1815, -23.3522) -> (33.1346, -23.3068) construction
  line L745 (33.0893, -23.2597) -> (33.0464, -23.2101) construction
  line L746 (33.0464, -23.2101) -> (33.014, -23.153) construction
  arc A126 (33.014, -23.153) -> (33.3939, -22.6017) centre (0, 0) ccw
  arc A127 (33.3939, -22.6017) -> (33.7646, -22.0441) centre (0, 0) ccw
  spline S243 degree 4 poles (34.0118, -22.1255) (33.9521, -22.0988) (33.8916, -22.0743) (33.8296, -22.0529) (33.7646, -22.0441) knots 1 1 1 1 1 2 2 2 2 2
  line L747 (34.0118, -22.1255) -> (33.9521, -22.0988) construction
  line L748 (33.9521, -22.0988) -> (33.8916, -22.0743) construction
  line L749 (33.8916, -22.0743) -> (33.8296, -22.0529) construction
  line L750 (33.8296, -22.0529) -> (33.7646, -22.0441) construction
  line L751 (38.5636, -19.4258) -> (37.2511, -19.2043) construction
  spline S244 degree 2 poles (38.5636, -19.4258) (37.2511, -19.2043) (35.9609, -18.7923) knots 1 1 1 2 2 2
  line L752 (37.2511, -19.2043) -> (35.9609, -18.7923) construction
  spline S245 degree 2 poles (37.1911, -21.9393) (36.2951, -20.955) (35.251, -20.0924) knots 1 1 1 2 2 2
  line L753 (37.1911, -21.9393) -> (36.2951, -20.955) construction
  line L754 (36.2951, -20.955) -> (35.251, -20.0924) construction
  line L755 (35.2, -20.0516) -> (35.1505, -20.009) construction
  spline S246 degree 4 poles (35.251, -20.0924) (35.2, -20.0516) (35.1505, -20.009) (35.103, -19.9637) (35.0654, -19.91) knots 1 1 1 1 1 2 2 2 2 2
  line L756 (35.251, -20.0924) -> (35.2, -20.0516) construction
  line L757 (35.1505, -20.009) -> (35.103, -19.9637) construction
  line L758 (35.103, -19.9637) -> (35.0654, -19.91) construction
  arc A128 (35.0654, -19.91) -> (35.3911, -19.325) centre (0, 0) ccw
  arc A129 (35.3911, -19.325) -> (35.7071, -18.7347) centre (0, 0) ccw
  spline S247 degree 4 poles (35.9609, -18.7923) (35.899, -18.7714) (35.8364, -18.7528) (35.7727, -18.7373) (35.7071, -18.7347) knots 1 1 1 1 1 2 2 2 2 2
  line L759 (35.9609, -18.7923) -> (35.899, -18.7714) construction
  line L760 (35.899, -18.7714) -> (35.8364, -18.7528) construction
  line L761 (35.8364, -18.7528) -> (35.7727, -18.7373) construction
  line L762 (35.7727, -18.7373) -> (35.7071, -18.7347) construction
  line L763 (40.2355, -15.6722) -> (38.9079, -15.5764) construction
  spline S248 degree 2 poles (40.2355, -15.6722) (38.9079, -15.5764) (37.5844, -15.2889) knots 1 1 1 2 2 2
  line L764 (38.9079, -15.5764) -> (37.5844, -15.2889) construction
  spline S249 degree 2 poles (39.1082, -18.3048) (38.1227, -17.41) (37.0013, -16.6506) knots 1 1 1 2 2 2
  line L765 (39.1082, -18.3048) -> (38.1227, -17.41) construction
  line L766 (38.1227, -17.41) -> (37.0013, -16.6506) construction
  line L767 (36.9466, -16.6148) -> (36.8933, -16.5772) construction
  spline S250 degree 4 poles (37.0013, -16.6506) (36.9466, -16.6148) (36.8933, -16.5772) (36.8417, -16.5366) (36.7992, -16.4867) knots 1 1 1 1 1 2 2 2 2 2
  line L768 (37.0013, -16.6506) -> (36.9466, -16.6148) construction
  line L769 (36.8933, -16.5772) -> (36.8417, -16.5366) construction
  line L770 (36.8417, -16.5366) -> (36.7992, -16.4867) construction
  arc A130 (36.7992, -16.4867) -> (37.0678, -15.8734) centre (0, 0) ccw
  arc A131 (37.0678, -15.8734) -> (37.3263, -15.2557) centre (0, 0) ccw
  spline S251 degree 4 poles (37.5844, -15.2889) (37.5208, -15.274) (37.4567, -15.2614) (37.3918, -15.252) (37.3263, -15.2557) knots 1 1 1 1 1 2 2 2 2 2
  line L771 (37.5844, -15.2889) -> (37.5208, -15.274) construction
  line L772 (37.5208, -15.274) -> (37.4567, -15.2614) construction
  line L773 (37.4567, -15.2614) -> (37.3918, -15.252) construction
  line L774 (37.3918, -15.252) -> (37.3263, -15.2557) construction
  line L775 (41.543, -11.7766) -> (40.2124, -11.8074) construction
  spline S252 degree 2 poles (41.543, -11.7766) (40.2124, -11.8074) (38.8675, -11.647) knots 1 1 1 2 2 2
  line L776 (40.2124, -11.8074) -> (38.8675, -11.647) construction
  spline S253 degree 2 poles (40.6711, -14.5044) (39.605, -13.7074) (38.4165, -13.058) knots 1 1 1 2 2 2
  line L777 (40.6711, -14.5044) -> (39.605, -13.7074) construction
  line L778 (39.605, -13.7074) -> (38.4165, -13.058) construction
  line L779 (38.3587, -13.0276) -> (38.302, -12.9952) construction
  spline S254 degree 4 poles (38.4165, -13.058) (38.3587, -13.0276) (38.302, -12.9952) (38.2468, -12.9597) (38.1997, -12.914) knots 1 1 1 1 1 2 2 2 2 2
  line L780 (38.4165, -13.058) -> (38.3587, -13.0276) construction
  line L781 (38.302, -12.9952) -> (38.2468, -12.9597) construction
  line L782 (38.2468, -12.9597) -> (38.1997, -12.914) construction
  arc A132 (38.1997, -12.914) -> (38.4088, -12.278) centre (0, 0) ccw
  arc A133 (38.4088, -12.278) -> (38.6074, -11.6385) centre (0, 0) ccw
  spline S255 degree 4 poles (38.8675, -11.647) (38.8028, -11.6382) (38.7378, -11.6318) (38.6723, -11.6287) (38.6074, -11.6385) knots 1 1 1 1 1 2 2 2 2 2
  line L783 (38.8675, -11.647) -> (38.8028, -11.6382) construction
  line L784 (38.8028, -11.6382) -> (38.7378, -11.6318) construction
  line L785 (38.7378, -11.6318) -> (38.6723, -11.6287) construction
  line L786 (38.6723, -11.6287) -> (38.6074, -11.6385) construction
  line L787 (42.4744, -7.7743) -> (41.1526, -7.9315) construction
  spline S256 degree 2 poles (42.4744, -7.7743) (41.1526, -7.9315) (39.7986, -7.8997) knots 1 1 1 2 2 2
  line L788 (41.1526, -7.9315) -> (39.7986, -7.8997) construction
  spline S257 degree 2 poles (41.8656, -10.5727) (40.7286, -9.8807) (39.4838, -9.3471) knots 1 1 1 2 2 2
  line L789 (41.8656, -10.5727) -> (40.7286, -9.8807) construction
  line L790 (40.7286, -9.8807) -> (39.4838, -9.3471) construction
  line L791 (39.4233, -9.3224) -> (39.3638, -9.2955) construction
  spline S258 degree 4 poles (39.4838, -9.3471) (39.4233, -9.3224) (39.3638, -9.2955) (39.3055, -9.2654) (39.2543, -9.2244) knots 1 1 1 1 1 2 2 2 2 2
  line L792 (39.4838, -9.3471) -> (39.4233, -9.3224) construction
  line L793 (39.3638, -9.2955) -> (39.3055, -9.2654) construction
  line L794 (39.3055, -9.2654) -> (39.2543, -9.2244) construction
  arc A134 (39.2543, -9.2244) -> (39.402, -8.5714) centre (0, 0) ccw
  arc A135 (39.402, -8.5714) -> (39.5389, -7.916) centre (0, 0) ccw
  spline S259 degree 4 poles (39.7986, -7.8997) (39.7334, -7.8971) (39.6681, -7.8968) (39.6025, -7.9) (39.5389, -7.916) knots 1 1 1 1 1 2 2 2 2 2
  line L795 (39.7986, -7.8997) -> (39.7334, -7.8971) construction
  line L796 (39.7334, -7.8971) -> (39.6681, -7.8968) construction
  line L797 (39.6681, -7.8968) -> (39.6025, -7.9) construction
  line L798 (39.6025, -7.9) -> (39.5389, -7.916) construction
  line L799 (43.021, -3.7017) -> (41.7202, -3.9838) construction
  spline S260 degree 2 poles (43.021, -3.7017) (41.7202, -3.9838) (40.3693, -4.0808) knots 1 1 1 2 2 2
  line L800 (41.7202, -3.9838) -> (40.3693, -4.0808) construction
  spline S261 degree 2 poles (42.6811, -6.5452) (41.4834, -5.9644) (40.1935, -5.5517) knots 1 1 1 2 2 2
  line L801 (42.6811, -6.5452) -> (41.4834, -5.9644) construction
  line L802 (41.4834, -5.9644) -> (40.1935, -5.5517) construction
  line L803 (40.131, -5.5328) -> (40.0692, -5.5116) construction
  spline S262 degree 4 poles (40.1935, -5.5517) (40.131, -5.5328) (40.0692, -5.5116) (40.0083, -5.4872) (39.9534, -5.4513) knots 1 1 1 1 1 2 2 2 2 2
  line L804 (40.1935, -5.5517) -> (40.131, -5.5328) construction
  line L805 (40.0692, -5.5116) -> (40.0083, -5.4872) construction
  line L806 (40.0083, -5.4872) -> (39.9534, -5.4513) construction
  arc A136 (39.9534, -5.4513) -> (40.0384, -4.7872) centre (0, 0) ccw
  arc A137 (40.0384, -4.7872) -> (40.1123, -4.1217) centre (0, 0) ccw
  spline S263 degree 4 poles (40.3693, -4.0808) (40.3041, -4.0844) (40.2391, -4.0904) (40.1742, -4.0997) (40.1123, -4.1217) knots 1 1 1 1 1 2 2 2 2 2
  line L807 (40.3693, -4.0808) -> (40.3041, -4.0844) construction
  line L808 (40.3041, -4.0844) -> (40.2391, -4.0904) construction
  line L809 (40.2391, -4.0904) -> (40.1742, -4.0997) construction
  line L810 (40.1742, -4.0997) -> (40.1123, -4.1217) construction
  point P0 (40.2208, 2.8766)
  point P1 (37.7811, 14.0916)
  point P2 (36.2706, 17.6192)
  point P3 (34.4315, 20.9871)
  point P4 (27.1241, 29.8375)
  point P5 (24.165, 32.2807)
  point P6 (17.6192, 36.2706)
  point P7 (14.0916, 37.7811)
  point P8 (10.4365, 38.9496)
  point P9 (6.6869, 39.7652)
  point P10 (2.8766, 40.2208)
  point P11 (-0.9596, 40.3121)
  point P12 (-4.7872, 40.0384)
  point P13 (-12.278, 38.4088)
  point P14 (-15.8734, 37.0678)
  point P15 (-19.325, 35.3911)
  point P16 (-25.6736, 31.0943)
  point P17 (-35.3911, 19.325)
  point P18 (-37.0678, 15.8734)
  point P19 (-38.4088, 12.278)
  point P20 (-40.0384, 4.7872)
  point P21 (-40.3121, 0.9596)
  point P22 (-40.2208, -2.8766)
  point P23 (-39.7652, -6.6869)
  point P24 (-38.9496, -10.4365)
  point P25 (-37.7811, -14.0916)
  point P26 (-36.2706, -17.6192)
  point P27 (-34.4315, -20.9871)
  point P28 (-27.1241, -29.8375)
  point P29 (-24.165, -32.2807)
  point P30 (-10.4365, -38.9496)
  point P31 (-6.6869, -39.7652)
  point P32 (-2.8766, -40.2208)
  point P33 (0.9596, -40.3121)
  point P34 (4.7872, -40.0384)
  point P35 (8.5714, -39.402)
  point P36 (12.278, -38.4088)
  point P37 (39.4442, 17.5689)
  point P38 (38.1929, 20.1449)
  point P39 (40.9356, 13.7399)
  point P40 (39.9348, 16.4232)
  point P41 (42.0563, 9.7866)
  point P42 (41.3151, 12.5528)
  point P43 (42.7962, 5.7445)
  point P44 (42.3213, 8.5687)
  point P45 (43.1484, 1.6505)
  point P46 (42.9441, 4.507)
  point P47 (15.8734, -37.0678)
  point P48 (22.6017, -33.3939)
  point P49 (31.0943, -25.6736)
  point P50 (35.3911, -19.325)
  dimension "d1" = 14.5
  dimension "d2" = 10.4934
  dimension "d12" = 75.5
  dimension "d15" = 40.3225
  dimension "d16" = 75.5
  dimension "d17" = 40.3225
  dimension "d18" = 75.5
  dimension "d19" = 40.3225
  dimension "d20" = 75.5
  dimension "d21" = 40.3225